Autodesk Inventor part; units mm, degrees
(part 5 of 11)
  arc A1597 (6.6453, 29.3854) -> (6.7017, 29.3342) centre (6.6735, 29.3598) ccw
  line L798 (7.1127, 29.843) -> (7.6112, 30.2647)
  arc A1598 (7.6358, 30.2356) -> (7.5866, 30.2938) centre (7.6112, 30.2647) ccw
  arc A1599 (7.0881, 29.8721) -> (7.1373, 29.8139) centre (7.1127, 29.843) ccw
  line L799 (7.6112, 30.2647) -> (8.1605, 30.6178)
  arc A1600 (8.1811, 30.5857) -> (8.1399, 30.6498) centre (8.1605, 30.6178) ccw
  arc A1601 (7.5906, 30.2968) -> (7.6318, 30.2327) centre (7.6112, 30.2647) ccw
  line L800 (8.1605, 30.6178) -> (8.7512, 30.8961)
  arc A1602 (8.7674, 30.8616) -> (8.7349, 30.9305) centre (8.7511, 30.8961) ccw
  arc A1603 (8.1443, 30.6522) -> (8.1768, 30.5833) centre (8.1605, 30.6178) ccw
  line L801 (8.7512, 30.8961) -> (9.3731, 31.0949)
  arc A1604 (9.3847, 31.0586) -> (9.3615, 31.1312) centre (9.3731, 31.0949) ccw
  arc A1605 (8.7395, 30.9324) -> (8.7627, 30.8598) centre (8.7511, 30.8961) ccw
  line L802 (9.3731, 31.0949) -> (10.0157, 31.2112)
  arc A1606 (10.0224, 31.1737) -> (10.0089, 31.2487) centre (10.0157, 31.2112) ccw
  arc A1607 (9.3663, 31.1324) -> (9.3798, 31.0574) centre (9.3731, 31.0949) ccw
  line L803 (10.0157, 31.2112) -> (10.6676, 31.2441)
  arc A1608 (10.6694, 31.206) -> (10.6658, 31.2821) centre (10.6676, 31.2441) ccw
  arc A1609 (10.0138, 31.2493) -> (10.0175, 31.1731) centre (10.0157, 31.2112) ccw
  line L804 (10.6676, 31.2441) -> (11.2768, 31.2186)
  arc A1610 (11.2731, 31.1809) -> (11.2777, 31.257) centre (11.2754, 31.2189) ccw
  arc A1611 (10.6699, 31.2821) -> (10.6653, 31.2061) centre (10.6676, 31.2441) ccw
  line L805 (11.2768, 31.2186) -> (11.8753, 31.0912)
  arc A1612 (11.8769, 31.0569) -> (11.8906, 31.1319) centre (11.8837, 31.0944) ccw
  arc A1613 (11.2822, 31.2564) -> (11.2685, 31.1815) centre (11.2754, 31.2189) ccw
  line L806 (11.8753, 31.0912) -> (12.4777, 30.9778)
  arc A1614 (12.4664, 30.9414) -> (12.489, 31.0142) centre (12.4777, 30.9778) ccw
  arc A1615 (11.8867, 31.1275) -> (11.864, 31.0548) centre (11.8753, 31.0912) ccw
  line L807 (12.4777, 30.9778) -> (12.9624, 30.6072)
  arc A1616 (12.9467, 30.5724) -> (12.978, 30.6419) centre (12.9624, 30.6072) ccw
  arc A1617 (12.4933, 31.0126) -> (12.462, 30.9431) centre (12.4777, 30.9778) ccw
  line L808 (12.9624, 30.6072) -> (14.3509, 26.7983)
  arc A1618 (14.3312, 26.7657) -> (14.3707, 26.8309) centre (14.3509, 26.7983) ccw
  arc A1619 (12.9821, 30.6398) -> (12.9427, 30.5746) centre (12.9624, 30.6072) ccw
  line L809 (14.3509, 26.7983) -> (23.3981, 15.1516)
  arc A1620 (23.4282, 15.1749) -> (23.4216, 15.1816) centre (23.3981, 15.1516) ccw
  arc A1621 (14.3744, 26.8283) -> (14.3274, 26.7683) centre (14.3509, 26.7983) ccw
  line L810 (23.3981, 15.1516) -> (19.5097, 19.7125)
  arc A1622 (16.8769, 22.7269) -> (16.8787, 22.7253) centre (16.8517, 22.6983) ccw
  arc A1623 (23.3654, 15.132) -> (23.3711, 15.1246) centre (23.3981, 15.1516) ccw
  line L811 (19.5097, 19.7125) -> (16.4438, 23.1565)
  arc A1624 (16.4139, 23.1331) -> (16.4738, 23.18) centre (16.4438, 23.1565) ccw
  arc A1625 (16.8233, 22.673) -> (16.8217, 22.6748) centre (16.8517, 22.6983) ccw
  line L812 (16.4438, 23.1565) -> (16.0942, 23.6606)
  arc A1626 (16.0616, 23.6409) -> (16.1268, 23.6803) centre (16.0942, 23.6606) ccw
  arc A1627 (16.4765, 23.1763) -> (16.4112, 23.1368) centre (16.4438, 23.1565) ccw
  line L813 (16.0942, 23.6606) -> (15.8078, 24.2031)
  arc A1628 (15.7731, 24.1874) -> (15.8426, 24.2187) centre (15.8078, 24.2031) ccw
  arc A1629 (16.1289, 23.6762) -> (16.0594, 23.6449) centre (16.0942, 23.6606) ccw
  line L814 (15.8078, 24.2031) -> (15.5889, 24.7761)
  arc A1630 (15.5525, 24.7648) -> (15.6253, 24.7875) centre (15.5889, 24.7761) ccw
  arc A1631 (15.8442, 24.2144) -> (15.7714, 24.1917) centre (15.8078, 24.2031) ccw
  line L815 (15.5889, 24.7761) -> (15.4407, 25.3714)
  arc A1632 (15.4032, 25.3645) -> (15.4781, 25.3783) centre (15.4407, 25.3714) ccw
  arc A1633 (15.6379, 27.3846) -> (15.5629, 27.3709) centre (15.6004, 27.3777) ccw
  line L816 (15.4407, 25.3714) -> (14.9039, 25.4351)
  arc A1634 (14.8659, 25.4328) -> (14.942, 25.4374) centre (14.9039, 25.4351) ccw
  arc A1635 (15.4787, 25.3737) -> (15.4026, 25.3691) centre (15.4407, 25.3714) ccw
  line L817 (14.9039, 25.4351) -> (18.8583, 22.6449)
  arc A1636 (18.8203, 22.6472) -> (18.8963, 22.6426) centre (18.8583, 22.6449) ccw
  arc A1637 (14.942, 25.4328) -> (14.8659, 25.4374) centre (14.9039, 25.4351) ccw
  line L818 (18.8583, 22.6449) -> (13.5985, 27.0666)
  arc A1638 (15.5629, 24.9531) -> (15.6379, 24.9394) centre (15.6004, 24.9463) ccw
  arc A1639 (18.8958, 22.638) -> (18.8208, 22.6517) centre (18.8583, 22.6449) ccw
  line L819 (13.5985, 27.0666) -> (5.328, 28.9324)
  arc A1640 (5.2916, 28.9437) -> (5.3643, 28.9211) centre (5.328, 28.9324) ccw
  arc A1641 (13.6349, 27.0553) -> (13.5621, 27.0779) centre (13.5985, 27.0666) ccw
  line L820 (5.328, 28.9324) -> (19.749, 27.0115)
  arc A1642 (5.9013, 28.867) -> (5.9708, 28.8358) centre (5.936, 28.8514) ccw
  arc A1643 (5.3627, 28.9167) -> (5.2932, 28.948) centre (5.328, 28.9324) ccw
  line L821 (19.749, 27.0115) -> (10.434, 29.4468)
  arc A1644 (10.4014, 29.4665) -> (10.4666, 29.4271) centre (10.434, 29.4468) ccw
  arc A1645 (19.7816, 26.9918) -> (19.7164, 27.0312) centre (19.749, 27.0115) ccw
  line L822 (10.434, 29.4468) -> (20.7175, 25.3208)
  arc A1646 (10.9892, 29.183) -> (11.0176, 29.2538) centre (11.0034, 29.2184) ccw
  arc A1647 (10.464, 29.4233) -> (10.404, 29.4703) centre (10.434, 29.4468) ccw
  line L823 (20.7175, 25.3208) -> (12.0354, 22.6782)
  arc A1648 (12.0377, 22.6402) -> (12.0332, 22.7163) centre (12.0354, 22.6782) ccw
  arc A1649 (11.0303, 29.1914) -> (10.9764, 29.2453) centre (11.0034, 29.2184) ccw
  line L824 (12.0354, 22.6782) -> (14.4431, 22.5281)
  arc A1650 (14.4196, 22.5581) -> (14.4666, 22.4982) centre (14.4431, 22.5281) ccw
  arc A1651 (12.0589, 22.6482) -> (12.0119, 22.7082) centre (12.0354, 22.6782) ccw
  line L825 (14.4431, 22.5281) -> (13.0207, 21.6798)
  arc A1652 (13.001, 21.7124) -> (13.0404, 21.6472) centre (13.0207, 21.6798) ccw
  arc A1653 (14.4628, 22.4955) -> (14.4234, 22.5608) centre (14.4431, 22.5281) ccw
  line L826 (13.0207, 21.6798) -> (12.4691, 21.4111)
  arc A1654 (12.4535, 21.4459) -> (12.4848, 21.3764) centre (12.4691, 21.4111) ccw
  arc A1655 (13.0363, 21.645) -> (13.005, 21.7145) centre (13.0207, 21.6798) ccw
  line L827 (12.4691, 21.4111) -> (11.8832, 21.2297)
  arc A1656 (11.8719, 21.2661) -> (11.8946, 21.1933) centre (11.8832, 21.2297) ccw
  arc A1657 (12.4805, 21.3748) -> (12.4578, 21.4475) centre (12.4691, 21.4111) ccw
  line L828 (11.8832, 21.2297) -> (11.28, 21.1185)
  arc A1658 (11.2731, 21.156) -> (11.2868, 21.081) centre (11.28, 21.1185) ccw
  arc A1659 (11.8906, 21.1921) -> (11.8769, 21.2671) centre (11.8837, 21.2296) ccw
  line L829 (11.28, 21.1185) -> (10.668, 21.0819)
  arc A1660 (10.6657, 21.1199) -> (10.6703, 21.0439) centre (10.668, 21.0819) ccw
  arc A1661 (11.2823, 21.0805) -> (11.2777, 21.1565) centre (11.28, 21.1185) ccw
  line L830 (10.668, 21.0819) -> (10.0106, 21.1406)
  arc A1662 (10.014, 21.1786) -> (10.0072, 21.1027) centre (10.0106, 21.1406) ccw
  arc A1663 (10.6646, 21.044) -> (10.6714, 21.1199) centre (10.668, 21.0819) ccw
  line L831 (10.0106, 21.1406) -> (9.3659, 21.2818)
  arc A1664 (9.3741, 21.319) -> (9.3578, 21.2446) centre (9.3659, 21.2818) ccw
  arc A1665 (10.0025, 21.1034) -> (10.0188, 21.1778) centre (10.0106, 21.1406) ccw
  line L832 (9.3659, 21.2818) -> (8.7436, 21.502)
  arc A1666 (8.7565, 21.5379) -> (8.7308, 21.4661) centre (8.7436, 21.502) ccw
  arc A1667 (9.3532, 21.2459) -> (9.3787, 21.3177) centre (9.3659, 21.2818) ccw
  line L833 (8.7436, 21.502) -> (8.1556, 21.8016)
  arc A1668 (8.1727, 21.8355) -> (8.1383, 21.7675) centre (8.1555, 21.8015) ccw
  arc A1669 (8.7264, 21.468) -> (8.7608, 21.536) centre (8.7436, 21.502) ccw
  line L834 (8.1556, 21.8016) -> (7.6091, 22.1716)
  arc A1670 (7.6305, 22.2032) -> (7.5877, 22.1401) centre (7.6091, 22.1716) ccw
  arc A1671 (8.1341, 21.7699) -> (8.1768, 21.833) centre (8.1555, 21.8015) ccw
  line L835 (7.6091, 22.1716) -> (7.1138, 22.6078)
  arc A1672 (7.139, 22.6364) -> (7.0887, 22.5793) centre (7.1138, 22.6078) ccw
  arc A1673 (7.5839, 22.143) -> (7.6343, 22.2002) centre (7.6091, 22.1716) ccw
  line L836 (7.1138, 22.6078) -> (6.6776, 23.1031)
  arc A1674 (6.7062, 23.1283) -> (6.649, 23.0779) centre (6.6776, 23.1031) ccw
  arc A1675 (7.0853, 22.5827) -> (7.1424, 22.633) centre (7.1138, 22.6078) ccw
  line L837 (6.6776, 23.1031) -> (6.3075, 23.6495)
  arc A1676 (6.339, 23.6708) -> (6.2759, 23.6281) centre (6.3075, 23.6495) ccw
  arc A1677 (6.6461, 23.0817) -> (6.7092, 23.1245) centre (6.6776, 23.1031) ccw
  line L838 (6.3075, 23.6495) -> (6.0093, 24.2382)
  arc A1678 (6.0432, 24.2554) -> (5.9753, 24.221) centre (6.0093, 24.2382) ccw
  arc A1679 (6.2735, 23.6323) -> (6.3415, 23.6667) centre (6.3075, 23.6495) ccw
  line L839 (6.0093, 24.2382) -> (5.7878, 24.8599)
  arc A1680 (5.8237, 24.8727) -> (5.7519, 24.8472) centre (5.7878, 24.8599) ccw
  arc A1681 (5.9734, 24.2254) -> (6.0451, 24.251) centre (6.0093, 24.2382) ccw
  line L840 (5.7878, 24.8599) -> (5.6466, 25.5046)
  arc A1682 (5.6838, 25.5128) -> (5.6094, 25.4965) centre (5.6466, 25.5046) ccw
  arc A1683 (5.7506, 24.8518) -> (5.825, 24.8681) centre (5.7878, 24.8599) ccw
  line L841 (5.6466, 25.5046) -> (5.588, 26.162)
  arc A1684 (5.6259, 26.1654) -> (5.5501, 26.1586) centre (5.588, 26.162) ccw
  arc A1685 (5.6087, 25.5012) -> (5.6846, 25.508) centre (5.6466, 25.5046) ccw
  line L842 (5.588, 26.162) -> (6.858, 26.162)
  arc A1686 (6.858, 26.1239) -> (6.858, 26.2001) centre (6.858, 26.162) ccw
  arc A1687 (5.588, 26.2001) -> (5.588, 26.1239) centre (5.588, 26.162) ccw
  line L843 (6.858, 26.162) -> (6.8774, 25.6365)
  arc A1688 (6.8393, 25.6351) -> (6.9155, 25.638) centre (6.8774, 25.6366) ccw
  arc A1689 (6.8961, 26.1634) -> (6.8199, 26.1606) centre (6.858, 26.162) ccw
  line L844 (6.8774, 25.6365) -> (6.9714, 25.1192)
  arc A1690 (6.9339, 25.1124) -> (7.0089, 25.126) centre (6.9714, 25.1192) ccw
  arc A1691 (6.9149, 25.6434) -> (6.8399, 25.6297) centre (6.8774, 25.6366) ccw
  line L845 (6.9714, 25.1192) -> (7.1381, 24.6205)
  arc A1692 (7.1019, 24.6085) -> (7.1742, 24.6326) centre (7.1381, 24.6206) ccw
  arc A1693 (7.0075, 25.1313) -> (6.9353, 25.1072) centre (6.9714, 25.1192) ccw
  line L846 (7.1381, 24.6205) -> (7.374, 24.1506)
  arc A1694 (7.34, 24.1335) -> (7.4081, 24.1677) centre (7.374, 24.1506) ccw
  arc A1695 (7.1721, 24.6376) -> (7.104, 24.6035) centre (7.1381, 24.6206) ccw
  line L847 (7.374, 24.1506) -> (7.6744, 23.7191)
  arc A1696 (7.6431, 23.6973) -> (7.7057, 23.7409) centre (7.6744, 23.7191) ccw
  arc A1697 (7.4053, 24.1724) -> (7.3427, 24.1289) centre (7.374, 24.1506) ccw
  line L848 (7.6744, 23.7191) -> (8.0332, 23.3347)
  arc A1698 (8.0053, 23.3087) -> (8.061, 23.3607) centre (8.0332, 23.3347) ccw
  arc A1699 (7.7023, 23.7451) -> (7.6465, 23.6931) centre (7.6744, 23.7191) ccw
  line L849 (8.0332, 23.3347) -> (8.443, 23.0053)
  arc A1700 (8.4191, 22.9756) -> (8.4669, 23.035) centre (8.443, 23.0053) ccw
  arc A1701 (8.057, 23.3644) -> (8.0093, 23.305) centre (8.0332, 23.3347) ccw
  line L850 (8.443, 23.0053) -> (8.8955, 22.7376)
  arc A1702 (8.8761, 22.7048) -> (8.9149, 22.7704) centre (8.8955, 22.7376) ccw
  arc A1703 (8.4624, 23.0381) -> (8.4236, 22.9725) centre (8.443, 23.0053) ccw
  line L851 (8.8955, 22.7376) -> (9.3815, 22.537)
  arc A1704 (9.367, 22.5018) -> (9.3961, 22.5722) centre (9.3815, 22.537) ccw
  arc A1705 (8.91, 22.7728) -> (8.881, 22.7024) centre (8.8955, 22.7376) ccw
  line L852 (9.3815, 22.537) -> (9.8911, 22.4076)
  arc A1706 (9.8818, 22.3706) -> (9.9005, 22.4445) centre (9.8911, 22.4076) ccw
  arc A1707 (9.3909, 22.5739) -> (9.3721, 22.5) centre (9.3815, 22.537) ccw
  line L853 (9.8911, 22.4076) -> (10.414, 22.352)
  arc A1708 (10.41, 22.3141) -> (10.418, 22.3899) centre (10.414, 22.352) ccw
  arc A1709 (9.8952, 22.4455) -> (9.8871, 22.3697) centre (9.8911, 22.4076) ccw
  line L854 (10.414, 22.352) -> (10.6681, 22.3519)
  arc A1710 (10.6681, 22.3138) -> (10.6681, 22.39) centre (10.6681, 22.3519) ccw
  arc A1711 (10.414, 22.3901) -> (10.414, 22.3139) centre (10.414, 22.352) ccw
  line L855 (10.6681, 22.3519) -> (11.2103, 22.3905)
  arc A1712 (11.213, 22.3525) -> (11.2076, 22.4285) centre (11.2103, 22.3905) ccw
  arc A1713 (10.6653, 22.3899) -> (10.6708, 22.3139) centre (10.6681, 22.3519) ccw
  line L856 (11.2103, 22.3905) -> (11.7415, 22.5058)
  arc A1714 (11.7496, 22.4686) -> (11.7334, 22.543) centre (11.7415, 22.5058) ccw
  arc A1715 (11.2022, 22.4277) -> (11.2184, 22.3532) centre (11.2103, 22.3905) ccw
  line L857 (11.7415, 22.5058) -> (12.2509, 22.6955)
  arc A1716 (12.264, 22.6606) -> (12.2374, 22.732) centre (12.2507, 22.6963) ccw
  arc A1717 (11.7282, 22.5415) -> (11.7548, 22.4701) centre (11.7415, 22.5058) ccw
  line L858 (12.2509, 22.6955) -> (12.7282, 22.9558)
  arc A1718 (12.7464, 22.9224) -> (12.7099, 22.9893) centre (12.7282, 22.9558) ccw
  arc A1719 (12.2325, 22.7297) -> (12.269, 22.6629) centre (12.2507, 22.6963) ccw
  line L859 (12.7282, 22.9558) -> (12.9175, 23.4562)
  arc A1720 (13.1859, 23.2521) -> (13.1402, 23.3131) centre (13.163, 23.2826) ccw
  arc A1721 (12.7053, 22.9863) -> (12.751, 22.9253) centre (12.7282, 22.9558) ccw
  line L860 (12.9175, 23.4562) -> (13.0355, 23.9868)
  arc A1722 (13.5743, 23.64) -> (13.5205, 23.6939) centre (13.5474, 23.667) ccw
  arc A1723 (13.1361, 23.3095) -> (13.19, 23.2557) centre (13.163, 23.2826) ccw
  line L861 (13.0355, 23.9868) -> (13.0769, 24.5288)
  arc A1724 (13.1074, 24.506) -> (13.0464, 24.5517) centre (13.0769, 24.5288) ccw
  arc A1725 (13.5169, 23.6898) -> (13.5779, 23.6441) centre (13.5474, 23.667) ccw
  line L862 (13.0769, 24.5288) -> (13.0407, 25.0712)
  arc A1726 (14.1671, 24.561) -> (14.1003, 24.5975) centre (14.1337, 24.5793) ccw
  arc A1727 (13.0435, 24.5471) -> (13.1103, 24.5106) centre (13.0769, 24.5288) ccw
  line L863 (13.0407, 25.0712) -> (12.9277, 25.6029)
  arc A1728 (12.9633, 25.5896) -> (12.892, 25.6162) centre (12.9277, 25.6029) ccw
  arc A1729 (14.098, 24.5926) -> (14.1694, 24.566) centre (14.1337, 24.5793) ccw
  line L864 (12.9277, 25.6029) -> (22.6056, 27.554)
  arc A1730 (22.6429, 27.5459) -> (22.5684, 27.5621) centre (22.6056, 27.554) ccw
  arc A1731 (12.8904, 25.611) -> (12.9649, 25.5948) centre (12.9277, 25.6029) ccw
  line L865 (22.6056, 27.554) -> (9.5434, 30.1539)
  arc A1732 (9.5814, 30.1512) -> (9.5054, 30.1566) centre (9.5434, 30.1539) ccw
  arc A1733 (22.5676, 27.5568) -> (22.6436, 27.5513) centre (22.6056, 27.554) ccw
  line L866 (9.5434, 30.1539) -> (9.9852, 30.1292)
  arc A1734 (10.0232, 30.1319) -> (9.9472, 30.1265) centre (9.9852, 30.1292) ccw
  arc A1735 (9.5054, 30.1512) -> (9.5814, 30.1566) centre (9.5434, 30.1539) ccw
  line L867 (9.9852, 30.1292) -> (10.4403, 29.8319)
  arc A1736 (10.4775, 29.84) -> (10.403, 29.8238) centre (10.4403, 29.8319) ccw
  arc A1737 (9.9479, 30.1211) -> (10.0224, 30.1373) centre (9.9852, 30.1292) ccw
  line L868 (10.4403, 29.8319) -> (10.9331, 29.6024)
  arc A1738 (14.1694, 27.758) -> (14.098, 27.7314) centre (14.1337, 27.7447) ccw
  arc A1739 (10.4046, 29.8186) -> (10.476, 29.8452) centre (10.4403, 29.8319) ccw
  line L869 (10.9331, 29.6024) -> (11.4535, 29.4454)
  arc A1740 (11.4869, 29.4637) -> (11.42, 29.4271) centre (11.4535, 29.4454) ccw
  arc A1741 (14.1003, 27.7265) -> (14.1671, 27.763) centre (14.1337, 27.7447) ccw
  line L870 (11.4535, 29.4454) -> (11.991, 29.364)
  arc A1742 (13.5779, 28.6799) -> (13.5169, 28.6342) centre (13.5474, 28.657) ccw
  arc A1743 (11.423, 29.4226) -> (11.484, 29.4682) centre (11.4535, 29.4454) ccw
  line L871 (11.991, 29.364) -> (12.5346, 29.36)
  arc A1744 (13.19, 29.0683) -> (13.1361, 29.0145) centre (13.163, 29.0414) ccw
  arc A1745 (13.5205, 28.6301) -> (13.5743, 28.684) centre (13.5474, 28.657) ccw
  line L872 (12.5346, 29.36) -> (12.7342, 29.3872)
  arc A1746 (12.7571, 29.4177) -> (12.7114, 29.3567) centre (12.7342, 29.3872) ccw
  arc A1747 (13.1402, 29.0109) -> (13.1859, 29.0719) centre (13.163, 29.0414) ccw
  line L873 (12.7342, 29.3872) -> (12.2551, 29.6441)
  arc A1748 (12.269, 29.6611) -> (12.2325, 29.5943) centre (12.2507, 29.6277) ccw
  arc A1749 (12.716, 29.3537) -> (12.7525, 29.4206) centre (12.7342, 29.3872) ccw
  line L874 (12.2551, 29.6441) -> (11.7444, 29.8301)
  arc A1750 (11.7577, 29.8658) -> (11.7311, 29.7945) centre (11.7444, 29.8301) ccw
  arc A1751 (12.2374, 29.592) -> (12.264, 29.6634) centre (12.2507, 29.6277) ccw
  line L875 (11.7444, 29.8301) -> (11.2123, 29.9416)
  arc A1752 (11.2204, 29.9789) -> (11.2042, 29.9044) centre (11.2123, 29.9416) ccw
  arc A1753 (11.7363, 29.7929) -> (11.7525, 29.8674) centre (11.7444, 29.8301) ccw
  line L876 (11.2123, 29.9416) -> (10.6698, 29.9763)
  arc A1754 (10.6726, 30.0143) -> (10.6671, 29.9383) centre (10.6698, 29.9763) ccw
  arc A1755 (11.2096, 29.9036) -> (11.2151, 29.9796) centre (11.2123, 29.9416) ccw
  line L877 (10.6698, 29.9763) -> (10.1821, 29.9523)
  arc A1756 (10.18, 29.9898) -> (10.1831, 29.9137) centre (10.1815, 29.9518) ccw
  arc A1757 (10.6714, 29.9382) -> (10.6683, 30.0144) centre (10.6698, 29.9763) ccw
  line L878 (10.1821, 29.9523) -> (9.7019, 29.8682)
  arc A1758 (9.6953, 29.9058) -> (9.7084, 29.8307) centre (9.7019, 29.8682) ccw
  arc A1759 (10.1881, 29.9142) -> (10.175, 29.9893) centre (10.1815, 29.9518) ccw
  line L879 (9.7019, 29.8682) -> (9.2372, 29.7228)
  arc A1760 (9.2258, 29.7591) -> (9.2486, 29.6864) centre (9.2372, 29.7228) ccw
  arc A1761 (9.7133, 29.8318) -> (9.6905, 29.9046) centre (9.7019, 29.8682) ccw
  line L880 (9.2372, 29.7228) -> (8.7955, 29.518)
  arc A1762 (8.7795, 29.5525) -> (8.8116, 29.4834) centre (8.7955, 29.5179) ccw
  arc A1763 (9.2533, 29.6882) -> (9.2212, 29.7573) centre (9.2372, 29.7228) ccw
  line L881 (8.7955, 29.518) -> (8.3843, 29.2572)
  arc A1764 (8.3639, 29.2894) -> (8.4047, 29.225) centre (8.3843, 29.2572) ccw
  arc A1765 (8.8159, 29.4857) -> (8.7751, 29.5501) centre (8.7955, 29.5179) ccw
  line L882 (8.3843, 29.2572) -> (8.0107, 28.945)
  arc A1766 (7.9863, 28.9742) -> (8.0352, 28.9157) centre (8.0107, 28.945) ccw
  arc A1767 (8.4088, 29.228) -> (8.3599, 29.2864) centre (8.3843, 29.2572) ccw
  line L883 (8.0107, 28.945) -> (7.6811, 28.5867)
  arc A1768 (7.653, 28.6125) -> (7.7091, 28.5609) centre (7.6811, 28.5867) ccw
  arc A1769 (8.0388, 28.9192) -> (7.9827, 28.9708) centre (8.0107, 28.945) ccw
  line L884 (7.6811, 28.5867) -> (7.401, 28.1884)
  arc A1770 (7.3698, 28.2104) -> (7.4321, 28.1665) centre (7.401, 28.1884) ccw
  arc A1771 (7.7122, 28.5648) -> (7.6499, 28.6086) centre (7.6811, 28.5867) ccw
  line L885 (7.401, 28.1884) -> (7.1753, 27.757)
  arc A1772 (7.1415, 27.7747) -> (7.209, 27.7394) centre (7.1753, 27.757) ccw
  arc A1773 (7.4347, 28.1708) -> (7.3672, 28.2061) centre (7.401, 28.1884) ccw
  line L886 (7.1753, 27.757) -> (7.6204, 27.5599)
  arc A1774 (6.972, 27.313) -> (7.0436, 27.2868) centre (7.0078, 27.2999) ccw
  arc A1775 (7.211, 27.7439) -> (7.1395, 27.7702) centre (7.1753, 27.757) ccw
  line L887 (7.6204, 27.5599) -> (6.9014, 26.8247)
  arc A1776 (6.8642, 26.8331) -> (6.9386, 26.8164) centre (6.9014, 26.8247) ccw
  arc A1777 (12.9568, 32.9698) -> (12.8825, 32.9865) centre (12.9197, 32.9781) ccw
  line L888 (6.9014, 26.8247) -> (6.858, 26.3398)
  arc A1778 (6.8201, 26.3432) -> (6.8959, 26.3364) centre (6.858, 26.3398) ccw
  arc A1779 (6.9394, 26.8213) -> (6.8635, 26.8281) centre (6.9014, 26.8247) ccw
  line L889 (6.858, 26.3398) -> (5.588, 26.3398)
  arc A1780 (5.588, 26.3779) -> (5.588, 26.3017) centre (5.588, 26.3398) ccw
  arc A1781 (6.858, 26.3017) -> (6.858, 26.3779) centre (6.858, 26.3398) ccw
  line L890 (15.4591, 25.2973) -> (14.7422, 26.1051)
  arc A1782 (14.7041, 26.1051) -> (14.7803, 26.1051) centre (14.7422, 26.1051) ccw
  arc A1783 (15.4972, 25.2973) -> (15.421, 25.2973) centre (15.4591, 25.2973) ccw
  line L891 (15.6556, 24.6016) -> (14.6713, 26.8246)
  arc A1784 (14.6332, 26.8246) -> (14.7094, 26.8246) centre (14.6713, 26.8246) ccw
  arc A1785 (15.6937, 24.6016) -> (15.6175, 24.6016) centre (15.6556, 24.6016) ccw
  line L892 (15.8368, 24.1482) -> (5.3895, 28.9242)
  arc A1786 (5.3514, 28.9242) -> (5.4276, 28.9242) centre (5.3895, 28.9242) ccw
  arc A1787 (15.8749, 24.1482) -> (15.7987, 24.1482) centre (15.8368, 24.1482) ccw
  line L893 (16.0101, 23.8198) -> (14.7162, 27.6819)
  arc A1788 (14.6781, 27.6819) -> (14.7543, 27.6819) centre (14.7162, 27.6819) ccw
  arc A1789 (16.0482, 23.8198) -> (15.972, 23.8198) centre (16.0101, 23.8198) ccw
  line L894 (16.1807, 23.5359) -> (19.6022, 27.0499)
  arc A1790 (19.5641, 27.0499) -> (19.6403, 27.0499) centre (19.6022, 27.0499) ccw
  arc A1791 (16.2188, 23.5359) -> (16.1426, 23.5359) centre (16.1807, 23.5359) ccw
  line L895 (16.3486, 23.2938) -> (14.8395, 28.295)
  arc A1792 (14.8014, 28.295) -> (14.8776, 28.295) centre (14.8395, 28.295) ccw
  arc A1793 (16.3867, 23.2938) -> (16.3105, 23.2938) centre (16.3486, 23.2938) ccw
  line L896 (16.515, 23.0767) -> (16.1422, 29.0049)
  arc A1794 (16.1041, 29.0049) -> (16.1803, 29.0049) centre (16.1422, 29.0049) ccw
  arc A1795 (16.5531, 23.0767) -> (16.4769, 23.0767) centre (16.515, 23.0767) ccw
  line L897 (16.6793, 22.8921) -> (10.7626, 29.315)
  arc A1796 (10.7245, 29.315) -> (10.8007, 29.315) centre (10.7626, 29.315) ccw
  arc A1797 (16.7174, 22.8921) -> (16.6412, 22.8921) centre (16.6793, 22.8921) ccw
  line L898 (12.0171, 28.1294) -> (9.5434, 30.1539)
  arc A1798 (9.5053, 30.1539) -> (9.5815, 30.1539) centre (9.5434, 30.1539) ccw
  arc A1799 (12.0552, 28.1294) -> (11.979, 28.1294) centre (12.0171, 28.1294) ccw
  line L899 (9.5434, 30.1539) -> (9.9028, 29.66)
  arc A1800 (9.8647, 29.66) -> (9.9409, 29.66) centre (9.9028, 29.66) ccw
  arc A1801 (9.5815, 30.1539) -> (9.5053, 30.1539) centre (9.5434, 30.1539) ccw
  line L900 (19.6426, 19.5567) -> (10.4327, 29.8369)
  arc A1802 (10.3946, 29.8369) -> (10.4708, 29.8369) centre (10.4327, 29.8369) ccw
  arc A1803 (19.6807, 19.5567) -> (19.6045, 19.5567) centre (19.6426, 19.5567) ccw
  line L901 (21.7522, 27.382) -> (20.5215, 25.2612)
  arc A1804 (20.4834, 25.2612) -> (20.5596, 25.2612) centre (20.5215, 25.2612) ccw
  arc A1805 (21.7903, 27.382) -> (21.7141, 27.382) centre (21.7522, 27.382) ccw
  line L902 (12.3669, 28.0907) -> (10.8306, 29.6501)
  arc A1806 (10.7925, 29.6501) -> (10.8687, 29.6501) centre (10.8306, 29.6501) ccw
  arc A1807 (12.405, 28.0907) -> (12.3288, 28.0907) centre (12.3669, 28.0907) ccw
  line L903 (13.0172, 25.1818) -> (14.192, 23.3346)
  arc A1808 (14.1539, 23.3346) -> (14.2301, 23.3346) centre (14.192, 23.3346) ccw
  arc A1809 (13.0553, 25.1818) -> (12.9791, 25.1818) centre (13.0172, 25.1818) ccw
  line L904 (12.58, 28.0916) -> (11.1586, 29.5344)
  arc A1810 (11.1205, 29.5344) -> (11.1967, 29.5344) centre (11.1586, 29.5344) ccw
  arc A1811 (12.6181, 28.0916) -> (12.5419, 28.0916) centre (12.58, 28.0916) ccw
  line L905 (13.0564, 24.8362) -> (14.1433, 23.1272)
  arc A1812 (14.1052, 23.1272) -> (14.1814, 23.1272) centre (14.1433, 23.1272) ccw
  arc A1813 (13.0945, 24.8362) -> (13.0183, 24.8362) centre (13.0564, 24.8362) ccw
  line L906 (23.5292, 14.9828) -> (11.4614, 29.4442)
  arc A1814 (11.4233, 29.4442) -> (11.4995, 29.4442) centre (11.4614, 29.4442) ccw
  arc A1815 (23.5673, 14.9828) -> (23.4911, 14.9828) centre (23.5292, 14.9828) ccw
  line L907 (13.0763, 24.5209) -> (12.2488, 22.6649)
  arc A1816 (12.2107, 22.6649) -> (12.2869, 22.6649) centre (12.2488, 22.6649) ccw
  arc A1817 (13.1144, 24.5209) -> (13.0382, 24.5209) centre (13.0763, 24.5209) ccw
  line L908 (23.648, 14.8299) -> (11.7128, 29.4061)
  arc A1818 (11.6747, 29.4061) -> (11.7509, 29.4061) centre (11.7128, 29.4061) ccw
  arc A1819 (23.6861, 14.8299) -> (23.6099, 14.8299) centre (23.648, 14.8299) ccw
  line L909 (13.0569, 24.2673) -> (12.442, 22.6529)
  arc A1820 (12.4039, 22.6529) -> (12.4801, 22.6529) centre (12.442, 22.6529) ccw
  arc A1821 (13.095, 24.2673) -> (13.0188, 24.2673) centre (13.0569, 24.2673) ccw
  line L910 (13.278, 28.1796) -> (11.9643, 29.3681)
  arc A1822 (11.9262, 29.3681) -> (12.0024, 29.3681) centre (11.9643, 29.3681) ccw
  arc A1823 (13.3161, 28.1796) -> (13.2399, 28.1796) centre (13.278, 28.1796) ccw
  line L911 (13.0376, 24.0137) -> (13.9419, 22.5594)
  arc A1824 (13.9038, 22.5594) -> (13.98, 22.5594) centre (13.9419, 22.5594) ccw
  arc A1825 (13.0757, 24.0137) -> (12.9995, 24.0137) centre (13.0376, 24.0137) ccw
  line L912 (14.2939, 26.9548) -> (13.2686, 25.6803)
  arc A1826 (13.2305, 25.6803) -> (13.3067, 25.6803) centre (13.2686, 25.6803) ccw
  arc A1827 (14.332, 26.9548) -> (14.2558, 26.9548) centre (14.2939, 26.9548) ccw
  line L913 (14.3098, 24.0785) -> (14.3, 22.4428)
  arc A1828 (14.2619, 22.4428) -> (14.3381, 22.4428) centre (14.3, 22.4428) ccw
  arc A1829 (14.3479, 24.0785) -> (14.2717, 24.0785) centre (14.3098, 24.0785) ccw
  line L914 (14.2329, 27.1221) -> (13.2454, 25.8946)
  arc A1830 (13.2073, 25.8946) -> (13.2835, 25.8946) centre (13.2454, 25.8946) ccw
  arc A1831 (14.271, 27.1221) -> (14.1948, 27.1221) centre (14.2329, 27.1221) ccw
  line L915 (14.1565, 23.927) -> (14.1471, 22.3516)
  arc A1832 (14.109, 22.3516) -> (14.1852, 22.3516) centre (14.1471, 22.3516) ccw
  arc A1833 (14.1946, 23.927) -> (14.1184, 23.927) centre (14.1565, 23.927) ccw
  line L916 (13.7852, 28.3501) -> (12.6046, 29.3695)
  arc A1834 (12.5665, 29.3695) -> (12.6427, 29.3695) centre (12.6046, 29.3695) ccw
  arc A1835 (13.8233, 28.3501) -> (13.7471, 28.3501) centre (13.7852, 28.3501) ccw
  line L917 (12.8925, 23.39) -> (13.6973, 22.0834)
  arc A1836 (13.6592, 22.0834) -> (13.7354, 22.0834) centre (13.6973, 22.0834) ccw
  arc A1837 (12.9306, 23.39) -> (12.8544, 23.39) centre (12.8925, 23.39) ccw
  line L918 (12.8972, 30.657) -> (12.5563, 29.2005)
  arc A1838 (12.5182, 29.2005) -> (12.5944, 29.2005) centre (12.5563, 29.2005) ccw
  arc A1839 (12.9353, 30.657) -> (12.8591, 30.657) centre (12.8972, 30.657) ccw
  line L919 (12.9015, 23.1391) -> (12.9469, 21.6439)
  arc A1840 (12.9088, 21.6439) -> (12.985, 21.6439) centre (12.9469, 21.6439) ccw
  arc A1841 (12.9396, 23.1391) -> (12.8634, 23.1391) centre (12.9015, 23.1391) ccw
  line L920 (12.7645, 30.7585) -> (12.4339, 29.3463)
  arc A1842 (12.3958, 29.3463) -> (12.472, 29.3463) centre (12.4339, 29.3463) ccw
  arc A1843 (12.8026, 30.7585) -> (12.7264, 30.7585) centre (12.7645, 30.7585) ccw
  line L921 (12.7526, 23.0204) -> (12.7967, 21.5707)
  arc A1844 (12.7586, 21.5707) -> (12.8348, 21.5707) centre (12.7967, 21.5707) ccw
  arc A1845 (12.7907, 23.0204) -> (12.7145, 23.0204) centre (12.7526, 23.0204) ccw
  line L922 (12.6444, 30.8503) -> (12.6553, 29.4295)
  arc A1846 (12.6172, 29.4295) -> (12.6934, 29.4295) centre (12.6553, 29.4295) ccw
  arc A1847 (12.6825, 30.8503) -> (12.6063, 30.8503) centre (12.6444, 30.8503) ccw
  line L923 (12.6495, 22.9129) -> (12.6464, 21.4975)
  arc A1848 (12.6083, 21.4975) -> (12.6845, 21.4975) centre (12.6464, 21.4975) ccw
  arc A1849 (12.6876, 22.9129) -> (12.6114, 22.9129) centre (12.6495, 22.9129) ccw
  line L924 (12.4915, 30.9178) -> (12.5022, 29.5116)
  arc A1850 (12.4641, 29.5116) -> (12.5403, 29.5116) centre (12.5022, 29.5116) ccw
  arc A1851 (12.5296, 30.9178) -> (12.4534, 30.9178) centre (12.4915, 30.9178) ccw
  line L925 (12.4971, 22.8298) -> (12.4962, 21.4243)
  arc A1852 (12.4581, 21.4243) -> (12.5343, 21.4243) centre (12.4962, 21.4243) ccw
  arc A1853 (12.5352, 22.8298) -> (12.459, 22.8298) centre (12.4971, 22.8298) ccw
  line L926 (12.3387, 30.9679) -> (12.3492, 29.5936)
  arc A1854 (12.3111, 29.5936) -> (12.3873, 29.5936) centre (12.3492, 29.5936) ccw
  arc A1855 (12.3768, 30.9679) -> (12.3006, 30.9679) centre (12.3387, 30.9679) ccw
  line L927 (12.3446, 22.7466) -> (12.344, 21.3723)
  arc A1856 (12.3059, 21.3723) -> (12.3821, 21.3723) centre (12.344, 21.3723) ccw
  arc A1857 (12.3827, 22.7466) -> (12.3065, 22.7466) centre (12.3446, 22.7466) ccw
  line L928 (12.1921, 31.0316) -> (12.1963, 29.6655)
  arc A1858 (12.1582, 29.6655) -> (12.2344, 29.6655) centre (12.1963, 29.6655) ccw
  arc A1859 (12.2302, 31.0316) -> (12.154, 31.0316) centre (12.1921, 31.0316) ccw
  line L929 (12.1922, 22.6736) -> (12.1916, 21.3252)
  arc A1860 (12.1535, 21.3252) -> (12.2297, 21.3252) centre (12.1916, 21.3252) ccw
  arc A1861 (12.2303, 22.6736) -> (12.1541, 22.6736) centre (12.1922, 22.6736) ccw
  line L930 (12.0334, 31.0614) -> (12.0434, 29.7212)
  arc A1862 (12.0053, 29.7212) -> (12.0815, 29.7212) centre (12.0434, 29.7212) ccw
  arc A1863 (12.0715, 31.0614) -> (11.9953, 31.0614) centre (12.0334, 31.0614) ccw
  line L931 (12.0398, 22.6169) -> (12.039, 21.2779)
  arc A1864 (12.0009, 21.2779) -> (12.0771, 21.2779) centre (12.039, 21.2779) ccw
  arc A1865 (12.0779, 22.6169) -> (12.0017, 22.6169) centre (12.0398, 22.6169) ccw
  line L932 (11.8805, 31.1069) -> (11.8906, 29.7769)
  arc A1866 (11.8525, 29.7769) -> (11.9287, 29.7769) centre (11.8906, 29.7769) ccw
  arc A1867 (11.9186, 31.1069) -> (11.8424, 31.1069) centre (11.8805, 31.1069) ccw
  line L933 (11.8874, 22.5601) -> (11.8867, 21.2301)
  arc A1868 (11.8486, 21.2301) -> (11.9248, 21.2301) centre (11.8867, 21.2301) ccw
  arc A1869 (11.9255, 22.5601) -> (11.8493, 22.5601) centre (11.8874, 22.5601) ccw
  line L934 (11.7348, 31.1217) -> (11.7348, 29.8191)
  arc A1870 (11.6967, 29.8191) -> (11.7729, 29.8191) centre (11.7348, 29.8191) ccw
  arc A1871 (11.7729, 31.1217) -> (11.6967, 31.1217) centre (11.7348, 31.1217) ccw
  line L935 (11.7348, 22.5049) -> (11.7348, 21.2023)
  arc A1872 (11.6967, 21.2023) -> (11.7729, 21.2023) centre (11.7348, 21.2023) ccw
  arc A1873 (11.7729, 22.5049) -> (11.6967, 22.5049) centre (11.7348, 22.5049) ccw
  line L936 (11.5757, 31.155) -> (11.5851, 29.8635)
  arc A1874 (11.547, 29.8635) -> (11.6232, 29.8635) centre (11.5851, 29.8635) ccw
  arc A1875 (11.6138, 31.155) -> (11.5376, 31.155) centre (11.5757, 31.155) ccw
  line L937 (11.5825, 22.4713) -> (11.582, 21.1742)
  arc A1876 (11.5439, 21.1742) -> (11.6201, 21.1742) centre (11.582, 21.1742) ccw
  arc A1877 (11.6206, 22.4713) -> (11.5444, 22.4713) centre (11.5825, 22.4713) ccw
  line L938 (11.4226, 31.1876) -> (11.4325, 29.8955)
  arc A1878 (11.3944, 29.8955) -> (11.4706, 29.8955) centre (11.4325, 29.8955) ccw
  arc A1879 (11.4607, 31.1876) -> (11.3845, 31.1876) centre (11.4226, 31.1876) ccw
  line L939 (11.4301, 22.4382) -> (11.4295, 21.1461)
  arc A1880 (11.3914, 21.1461) -> (11.4676, 21.1461) centre (11.4295, 21.1461) ccw
  arc A1881 (11.4682, 22.4382) -> (11.392, 22.4382) centre (11.4301, 22.4382) ccw
  line L940 (11.27, 31.214) -> (11.2798, 29.9275)
  arc A1882 (11.2417, 29.9275) -> (11.3179, 29.9275) centre (11.2798, 29.9275) ccw
  arc A1883 (11.3081, 31.214) -> (11.2319, 31.214) centre (11.27, 31.214) ccw
  line L941 (11.2777, 22.4051) -> (11.2771, 21.1186)
  arc A1884 (11.239, 21.1186) -> (11.3152, 21.1186) centre (11.2771, 21.1186) ccw
  arc A1885 (11.3158, 22.4051) -> (11.2396, 22.4051) centre (11.2777, 22.4051) ccw
  line L942 (11.1215, 31.2251) -> (11.1453, 29.9503)
  arc A1886 (11.1072, 29.9503) -> (11.1834, 29.9503) centre (11.1453, 29.9503) ccw
  arc A1887 (11.1596, 31.2251) -> (11.0834, 31.2251) centre (11.1215, 31.2251) ccw
  line L943 (11.1258, 22.3843) -> (11.1249, 21.1092)
  arc A1888 (11.0868, 21.1092) -> (11.163, 21.1092) centre (11.1249, 21.1092) ccw
  arc A1889 (11.1639, 22.3843) -> (11.0877, 22.3843) centre (11.1258, 22.3843) ccw
  line L944 (10.969, 31.2315) -> (10.9748, 29.9568)
  arc A1890 (10.9367, 29.9568) -> (11.0129, 29.9568) centre (10.9748, 29.9568) ccw
  arc A1891 (11.0071, 31.2315) -> (10.9309, 31.2315) centre (10.969, 31.2315) ccw
  line L945 (10.9729, 22.3736) -> (10.9725, 21.1001)
  arc A1892 (10.9344, 21.1001) -> (11.0106, 21.1001) centre (10.9725, 21.1001) ccw
  arc A1893 (11.011, 22.3736) -> (10.9348, 22.3736) centre (10.9729, 22.3736) ccw
  line L946 (10.8126, 31.238) -> (10.8223, 29.9665)
  arc A1894 (10.7842, 29.9665) -> (10.8604, 29.9665) centre (10.8223, 29.9665) ccw
  arc A1895 (10.8507, 31.238) -> (10.7745, 31.238) centre (10.8126, 31.238) ccw
  line L947 (10.8205, 22.3628) -> (10.8198, 21.091)
  arc A1896 (10.7817, 21.091) -> (10.8579, 21.091) centre (10.8198, 21.091) ccw
  arc A1897 (10.8586, 22.3628) -> (10.7824, 22.3628) centre (10.8205, 22.3628) ccw
  line L948 (10.6676, 31.2441) -> (10.6698, 29.9763)
  arc A1898 (10.6317, 29.9763) -> (10.7079, 29.9763) centre (10.6698, 29.9763) ccw
  arc A1899 (10.7057, 31.2441) -> (10.6295, 31.2441) centre (10.6676, 31.2441) ccw
  line L949 (10.6681, 22.3519) -> (10.668, 21.0819)
  arc A1900 (10.6299, 21.0819) -> (10.7061, 21.0819) centre (10.668, 21.0819) ccw
  arc A1901 (10.7062, 22.3519) -> (10.63, 22.352) centre (10.6681, 22.3519) ccw
  line L950 (10.5152, 31.2364) -> (10.5175, 29.9688)
  arc A1902 (10.4794, 29.9688) -> (10.5556, 29.9688) centre (10.5175, 29.9688) ccw
  arc A1903 (10.5533, 31.2364) -> (10.4771, 31.2364) centre (10.5152, 31.2364) ccw
  line L951 (10.5157, 22.352) -> (10.5156, 21.0955)
  arc A1904 (10.4775, 21.0955) -> (10.5537, 21.0955) centre (10.5156, 21.0955) ccw
  arc A1905 (10.5538, 22.352) -> (10.4776, 22.352) centre (10.5157, 22.352) ccw
  line L952 (10.3629, 31.2287) -> (10.3651, 29.9613)
  arc A1906 (10.327, 29.9613) -> (10.4032, 29.9613) centre (10.3651, 29.9613) ccw
  arc A1907 (10.401, 31.2287) -> (10.3248, 31.2287) centre (10.3629, 31.2287) ccw
  line L953 (10.3633, 22.3574) -> (10.3632, 21.1091)
  arc A1908 (10.3251, 21.1091) -> (10.4013, 21.1091) centre (10.3632, 21.1091) ccw
  arc A1909 (10.4014, 22.3574) -> (10.3252, 22.3574) centre (10.3633, 22.3574) ccw
  line L954 (10.2105, 31.221) -> (10.2142, 29.9538)
  arc A1910 (10.1761, 29.9538) -> (10.2523, 29.9538) centre (10.2142, 29.9538) ccw
  arc A1911 (10.2486, 31.221) -> (10.1724, 31.221) centre (10.2105, 31.221) ccw
  line L955 (10.2108, 22.3736) -> (10.2108, 21.1228)
  arc A1912 (10.1727, 21.1228) -> (10.2489, 21.1228) centre (10.2108, 21.1228) ccw
  arc A1913 (10.2489, 22.3736) -> (10.1727, 22.3736) centre (10.2108, 22.3736) ccw
  line L956 (10.0579, 31.2133) -> (10.059, 29.9307)
  arc A1914 (10.0209, 29.9307) -> (10.0971, 29.9307) centre (10.059, 29.9307) ccw
  arc A1915 (10.096, 31.2133) -> (10.0198, 31.2133) centre (10.0579, 31.2133) ccw
  line L957 (10.0584, 22.3898) -> (10.0584, 21.1364)
  arc A1916 (10.0203, 21.1364) -> (10.0965, 21.1364) centre (10.0584, 21.1364) ccw
  arc A1917 (10.0965, 22.3898) -> (10.0203, 22.3898) centre (10.0584, 22.3898) ccw
  line L958 (9.9059, 31.1913) -> (9.9066, 29.904)
  arc A1918 (9.8685, 29.904) -> (9.9447, 29.904) centre (9.9066, 29.904) ccw
  arc A1919 (9.944, 31.1913) -> (9.8678, 31.1913) centre (9.9059, 31.1913) ccw
  line L959 (9.906, 22.406) -> (9.906, 21.1635)
  arc A1920 (9.8679, 21.1635) -> (9.9441, 21.1635) centre (9.906, 21.1635) ccw
  arc A1921 (9.9441, 22.406) -> (9.8679, 22.406) centre (9.906, 22.406) ccw
  line L960 (9.7535, 31.1637) -> (9.7542, 29.8774)
  arc A1922 (9.7161, 29.8774) -> (9.7923, 29.8774) centre (9.7542, 29.8774) ccw
  arc A1923 (9.7916, 31.1637) -> (9.7154, 31.1637) centre (9.7535, 31.1637) ccw
  line L961 (9.7536, 22.4425) -> (9.7536, 21.1969)
  arc A1924 (9.7155, 21.1969) -> (9.7917, 21.1969) centre (9.7536, 21.1969) ccw
  arc A1925 (9.7917, 22.4425) -> (9.7155, 22.4425) centre (9.7536, 22.4425) ccw
  line L962 (9.6011, 31.1362) -> (9.6012, 29.8367)
  arc A1926 (9.5631, 29.8367) -> (9.6393, 29.8367) centre (9.6012, 29.8367) ccw
  arc A1927 (9.6392, 31.1362) -> (9.563, 31.1362) centre (9.6011, 31.1362) ccw
  line L963 (9.6012, 22.4812) -> (9.6012, 21.2303)
  arc A1928 (9.5631, 21.2303) -> (9.6393, 21.2303) centre (9.6012, 21.2303) ccw
  arc A1929 (9.6393, 22.4812) -> (9.5631, 22.4812) centre (9.6012, 22.4812) ccw
  line L964 (9.4488, 31.1086) -> (9.4488, 29.789)
  arc A1930 (9.4107, 29.789) -> (9.4869, 29.789) centre (9.4488, 29.789) ccw
  arc A1931 (9.4869, 31.1086) -> (9.4107, 31.1086) centre (9.4488, 31.1086) ccw
  line L965 (9.4488, 22.5199) -> (9.4488, 21.2637)
  arc A1932 (9.4107, 21.2637) -> (9.4869, 21.2637) centre (9.4488, 21.2637) ccw
  arc A1933 (9.4869, 22.5199) -> (9.4107, 22.5199) centre (9.4488, 22.5199) ccw
  line L966 (9.2963, 31.0703) -> (9.2964, 29.7413)
  arc A1934 (9.2583, 29.7413) -> (9.3345, 29.7413) centre (9.2964, 29.7413) ccw
  arc A1935 (9.3344, 31.0703) -> (9.2582, 31.0703) centre (9.2963, 31.0703) ccw
  line L967 (9.2935, 22.572) -> (9.2962, 21.3065)
  arc A1936 (9.2581, 21.3065) -> (9.3343, 21.3065) centre (9.2962, 21.3065) ccw
  arc A1937 (9.3316, 22.572) -> (9.2554, 22.572) centre (9.2935, 22.572) ccw
  line L968 (9.144, 31.0217) -> (9.144, 29.6795)
  arc A1938 (9.1059, 29.6795) -> (9.1821, 29.6795) centre (9.144, 29.6795) ccw
  arc A1939 (9.1821, 31.0217) -> (9.1059, 31.0217) centre (9.144, 31.0217) ccw
  line L969 (9.144, 22.635) -> (9.1437, 21.3604)
  arc A1940 (9.1056, 21.3604) -> (9.1818, 21.3604) centre (9.1437, 21.3604) ccw
  arc A1941 (9.1821, 22.635) -> (9.1059, 22.635) centre (9.144, 22.635) ccw
  line L970 (8.9917, 30.973) -> (8.9916, 29.6089)
  arc A1942 (8.9535, 29.6089) -> (9.0297, 29.6089) centre (8.9916, 29.6089) ccw
  arc A1943 (9.0298, 30.973) -> (8.9536, 30.973) centre (8.9917, 30.973) ccw
  line L971 (8.9885, 22.6972) -> (8.9912, 21.4144)
  arc A1944 (8.9531, 21.4144) -> (9.0293, 21.4144) centre (8.9912, 21.4144) ccw
  arc A1945 (9.0266, 22.6972) -> (8.9504, 22.6972) centre (8.9885, 22.6972) ccw
  line L972 (8.8391, 30.9242) -> (8.8392, 29.5382)
  arc A1946 (8.8011, 29.5382) -> (8.8773, 29.5382) centre (8.8392, 29.5382) ccw
  arc A1947 (8.8772, 30.9242) -> (8.801, 30.9242) centre (8.8391, 30.9242) ccw
  line L973 (8.8392, 22.7709) -> (8.8392, 21.4694)
  arc A1948 (8.8011, 21.4694) -> (8.8773, 21.4694) centre (8.8392, 21.4694) ccw
  arc A1949 (8.8773, 22.7709) -> (8.8011, 22.7709) centre (8.8392, 22.7709) ccw
  line L974 (8.6868, 30.8657) -> (8.6868, 29.449)
  arc A1950 (8.6487, 29.449) -> (8.7249, 29.449) centre (8.6868, 29.449) ccw
  arc A1951 (8.7249, 30.8657) -> (8.6487, 30.8657) centre (8.6868, 30.8657) ccw
  line L975 (8.6868, 22.8611) -> (8.6863, 21.5312)
  arc A1952 (8.6482, 21.5312) -> (8.7244, 21.5312) centre (8.6863, 21.5312) ccw
  arc A1953 (8.7249, 22.8611) -> (8.6487, 22.8611) centre (8.6868, 22.8611) ccw
  line L976 (8.5343, 30.7939) -> (8.5344, 29.3523)
  arc A1954 (8.4963, 29.3523) -> (8.5725, 29.3523) centre (8.5344, 29.3523) ccw
  arc A1955 (8.5724, 30.7939) -> (8.4962, 30.7939) centre (8.5343, 30.7939) ccw
  line L977 (8.5344, 22.9512) -> (8.5344, 21.6096)
  arc A1956 (8.4963, 21.6096) -> (8.5725, 21.6096) centre (8.5344, 21.6096) ccw
  arc A1957 (8.5725, 22.9512) -> (8.4963, 22.9512) centre (8.5344, 22.9512) ccw
  line L978 (8.3819, 30.7221) -> (8.382, 29.2552)
  arc A1958 (8.3439, 29.2552) -> (8.4201, 29.2552) centre (8.382, 29.2552) ccw
  arc A1959 (8.42, 30.7221) -> (8.3438, 30.7221) centre (8.3819, 30.7221) ccw
  line L979 (8.382, 23.0543) -> (8.3818, 21.6863)
  arc A1960 (8.3437, 21.6863) -> (8.4199, 21.6863) centre (8.3818, 21.6863) ccw
  arc A1961 (8.4201, 23.0543) -> (8.3439, 23.0543) centre (8.382, 23.0543) ccw
  line L980 (8.2296, 30.6503) -> (8.2296, 29.1279)
  arc A1962 (8.1915, 29.1279) -> (8.2677, 29.1279) centre (8.2296, 29.1279) ccw
  arc A1963 (8.2677, 30.6503) -> (8.1915, 30.6503) centre (8.2296, 30.6503) ccw
  line L981 (8.2296, 23.1768) -> (8.2296, 21.7639)
  arc A1964 (8.1915, 21.7639) -> (8.2677, 21.7639) centre (8.2296, 21.7639) ccw
  arc A1965 (8.2677, 23.1768) -> (8.1915, 23.1768) centre (8.2296, 23.1768) ccw
  line L982 (8.0772, 30.5642) -> (8.0772, 29.0005)
  arc A1966 (8.0391, 29.0005) -> (8.1153, 29.0005) centre (8.0772, 29.0005) ccw
  arc A1967 (8.1153, 30.5642) -> (8.0391, 30.5642) centre (8.0772, 30.5642) ccw
  line L983 (8.0772, 23.2993) -> (8.0773, 21.8546)
  arc A1968 (8.0392, 21.8546) -> (8.1154, 21.8546) centre (8.0773, 21.8546) ccw
  arc A1969 (8.1153, 23.2993) -> (8.0391, 23.2993) centre (8.0772, 23.2993) ccw
  line L984 (7.9248, 30.4662) -> (7.9248, 28.8516)
  arc A1970 (7.8867, 28.8516) -> (7.9629, 28.8516) centre (7.9248, 28.8516) ccw
  arc A1971 (7.9629, 30.4662) -> (7.8867, 30.4662) centre (7.9248, 30.4662) ccw
  line L985 (7.9248, 23.4508) -> (7.9249, 21.9578)
  arc A1972 (7.8868, 21.9578) -> (7.963, 21.9578) centre (7.9249, 21.9578) ccw
  arc A1973 (7.9629, 23.4508) -> (7.8867, 23.4508) centre (7.9248, 23.4508) ccw
  line L986 (7.7724, 30.3683) -> (7.7724, 28.6859)
  arc A1974 (7.7343, 28.6859) -> (7.8105, 28.6859) centre (7.7724, 28.6859) ccw
  arc A1975 (7.8105, 30.3683) -> (7.7343, 30.3683) centre (7.7724, 30.3683) ccw
  line L987 (7.7724, 23.6141) -> (7.7724, 22.061)
  arc A1976 (7.7343, 22.061) -> (7.8105, 22.061) centre (7.7724, 22.061) ccw
  arc A1977 (7.8105, 23.6141) -> (7.7343, 23.6141) centre (7.7724, 23.6141) ccw
  line L988 (7.62, 30.2703) -> (7.62, 28.4999)
  arc A1978 (7.5819, 28.4999) -> (7.6581, 28.4999) centre (7.62, 28.4999) ccw
  arc A1979 (7.6581, 30.2703) -> (7.5819, 30.2703) centre (7.62, 30.2703) ccw
  line L989 (7.62, 23.7973) -> (7.62, 22.1642)
  arc A1980 (7.5819, 22.1642) -> (7.6581, 22.1642) centre (7.62, 22.1642) ccw
  arc A1981 (7.6581, 23.7973) -> (7.5819, 23.7973) centre (7.62, 23.7973) ccw
  line L990 (7.4676, 30.1432) -> (7.4676, 28.2832)
  arc A1982 (7.4295, 28.2832) -> (7.5057, 28.2832) centre (7.4676, 28.2832) ccw
  arc A1983 (7.5057, 30.1432) -> (7.4295, 30.1432) centre (7.4676, 30.1432) ccw
  line L991 (7.4676, 24.0162) -> (7.4676, 22.2963)
  arc A1984 (7.4295, 22.2963) -> (7.5057, 22.2963) centre (7.4676, 22.2963) ccw
  arc A1985 (7.5057, 24.0162) -> (7.4295, 24.0162) centre (7.4676, 24.0162) ccw
  line L992 (7.3152, 30.0143) -> (7.3152, 28.0245)
  arc A1986 (7.2771, 28.0245) -> (7.3533, 28.0245) centre (7.3152, 28.0245) ccw
  arc A1987 (7.3533, 30.0143) -> (7.2771, 30.0143) centre (7.3152, 30.0143) ccw
  line L993 (7.3152, 24.2678) -> (7.3152, 22.4305)
  arc A1988 (7.2771, 22.4305) -> (7.3533, 22.4305) centre (7.3152, 22.4305) ccw
  arc A1989 (7.3533, 24.2678) -> (7.2771, 24.2678) centre (7.3152, 24.2678) ccw
  line L994 (7.1628, 29.8854) -> (7.2084, 27.7423)
  arc A1990 (7.1703, 27.7423) -> (7.2465, 27.7423) centre (7.2084, 27.7423) ccw
  arc A1991 (7.2009, 29.8854) -> (7.1247, 29.8854) centre (7.1628, 29.8854) ccw
  line L995 (7.1628, 24.5713) -> (7.1628, 22.5647)
  arc A1992 (7.1247, 22.5647) -> (7.2009, 22.5647) centre (7.1628, 22.5647) ccw
  arc A1993 (7.2009, 24.5713) -> (7.1247, 24.5713) centre (7.1628, 24.5713) ccw
  line L996 (7.0104, 29.7304) -> (7.6135, 27.563)
  arc A1994 (7.5754, 27.563) -> (7.6516, 27.563) centre (7.6135, 27.563) ccw
  arc A1995 (7.0485, 29.7304) -> (6.9723, 29.7304) centre (7.0104, 29.7304) ccw
  line L997 (7.0104, 25.0026) -> (7.0104, 22.7253)
  arc A1996 (6.9723, 22.7253) -> (7.0485, 22.7253) centre (7.0104, 22.7253) ccw
  arc A1997 (7.0485, 25.0026) -> (6.9723, 25.0026) centre (7.0104, 25.0026) ccw
  line L998 (6.858, 29.5628) -> (6.858, 26.3398)
  arc A1998 (6.8199, 26.3398) -> (6.8961, 26.3398) centre (6.858, 26.3398) ccw
  arc A1999 (6.8961, 29.5628) -> (6.8199, 29.5628) centre (6.858, 29.5628) ccw
  line L999 (6.858, 26.162) -> (6.858, 22.8983)
  arc A2000 (6.8199, 22.8983) -> (6.8961, 22.8983) centre (6.858, 22.8983) ccw
  arc A2001 (6.8961, 26.162) -> (6.8199, 26.162) centre (6.858, 26.162) ccw
  line L1000 (6.7056, 29.3951) -> (6.7056, 26.3398)
  arc A2002 (6.6675, 26.3398) -> (6.7437, 26.3398) centre (6.7056, 26.3398) ccw
  arc A2003 (6.7437, 29.3951) -> (6.6675, 29.3951) centre (6.7056, 29.3951) ccw
  line L1001 (6.7056, 26.162) -> (6.7056, 23.0713)
  arc A2004 (6.6675, 23.0713) -> (6.7437, 23.0713) centre (6.7056, 23.0713) ccw
  arc A2005 (6.7437, 26.162) -> (6.6675, 26.162) centre (6.7056, 26.162) ccw
  line L1002 (6.5532, 29.1865) -> (6.5532, 26.3398)
  arc A2006 (6.5151, 26.3398) -> (6.5913, 26.3398) centre (6.5532, 26.3398) ccw
  arc A2007 (6.5913, 29.1865) -> (6.5151, 29.1865) centre (6.5532, 29.1865) ccw
  line L1003 (6.5532, 26.162) -> (6.5532, 23.2868)
  arc A2008 (6.5151, 23.2868) -> (6.5913, 23.2868) centre (6.5532, 23.2868) ccw
  arc A2009 (6.5913, 26.162) -> (6.5151, 26.162) centre (6.5532, 26.162) ccw
  line L1004 (6.4008, 28.967) -> (6.4008, 26.3398)
  arc A2010 (6.3627, 26.3398) -> (6.4389, 26.3398) centre (6.4008, 26.3398) ccw
  arc A2011 (6.4389, 28.967) -> (6.3627, 28.967) centre (6.4008, 28.967) ccw
  line L1005 (6.4008, 26.162) -> (6.4008, 23.5117)
  arc A2012 (6.3627, 23.5117) -> (6.4389, 23.5117) centre (6.4008, 23.5117) ccw
  arc A2013 (6.4389, 26.162) -> (6.3627, 26.162) centre (6.4008, 26.162) ccw
  line L1006 (6.2484, 28.7212) -> (6.2484, 26.3398)
  arc A2014 (6.2103, 26.3398) -> (6.2865, 26.3398) centre (6.2484, 26.3398) ccw
  arc A2015 (6.2865, 28.7212) -> (6.2103, 28.7212) centre (6.2484, 28.7212) ccw
  line L1007 (6.2484, 26.162) -> (6.2484, 23.7661)
  arc A2016 (6.2103, 23.7661) -> (6.2865, 23.7661) centre (6.2484, 23.7661) ccw
  arc A2017 (6.2865, 26.162) -> (6.2103, 26.162) centre (6.2484, 26.162) ccw
  line L1008 (6.096, 28.4255) -> (6.096, 26.3398)
  arc A2018 (6.0579, 26.3398) -> (6.1341, 26.3398) centre (6.096, 26.3398) ccw
  arc A2019 (6.1341, 28.4255) -> (6.0579, 28.4255) centre (6.096, 28.4255) ccw
  line L1009 (6.096, 26.162) -> (6.096, 24.067)
  arc A2020 (6.0579, 24.067) -> (6.1341, 24.067) centre (6.096, 24.067) ccw
  arc A2021 (6.1341, 26.162) -> (6.0579, 26.162) centre (6.096, 26.162) ccw
  line L1010 (5.9436, 28.0807) -> (5.9436, 26.3398)
  arc A2022 (5.9055, 26.3398) -> (5.9817, 26.3398) centre (5.9436, 26.3398) ccw
  arc A2023 (5.9817, 28.0807) -> (5.9055, 28.0807) centre (5.9436, 28.0807) ccw
  line L1011 (5.9436, 26.162) -> (5.9436, 24.4226)
  arc A2024 (5.9055, 24.4226) -> (5.9817, 24.4226) centre (5.9436, 24.4226) ccw
  arc A2025 (5.9817, 26.162) -> (5.9055, 26.162) centre (5.9436, 26.162) ccw
  line L1012 (5.7912, 27.6567) -> (5.7912, 26.3398)
  arc A2026 (5.7531, 26.3398) -> (5.8293, 26.3398) centre (5.7912, 26.3398) ccw
  arc A2027 (5.8293, 27.6567) -> (5.7531, 27.6567) centre (5.7912, 27.6567) ccw
  line L1013 (5.7912, 26.162) -> (5.7912, 24.8504)
  arc A2028 (5.7531, 24.8504) -> (5.8293, 24.8504) centre (5.7912, 24.8504) ccw
  arc A2029 (5.8293, 26.162) -> (5.7531, 26.162) centre (5.7912, 26.162) ccw
  line L1014 (5.6388, 26.9485) -> (5.6388, 26.3398)
  arc A2030 (5.6007, 26.3398) -> (5.6769, 26.3398) centre (5.6388, 26.3398) ccw
  arc A2031 (5.6769, 26.9485) -> (5.6007, 26.9485) centre (5.6388, 26.9485) ccw
  line L1015 (5.6388, 26.162) -> (5.6388, 25.5924)
  arc A2032 (5.6007, 25.5924) -> (5.6769, 25.5924) centre (5.6388, 25.5924) ccw
  arc A2033 (5.6769, 26.162) -> (5.6007, 26.162) centre (5.6388, 26.162) ccw
  line L1016 (28.3443, 10.7495) -> (31.1877, 9.8395)
  arc A2034 (31.1497, 9.8426) -> (31.2257, 9.8363) centre (31.1877, 9.8395) ccw
  arc A2035 (28.3823, 10.7463) -> (28.3063, 10.7527) centre (28.3443, 10.7495) ccw
  line L1017 (31.1877, 9.8395) -> (31.0489, 9.2014)
  arc A2036 (31.0117, 9.2095) -> (31.0861, 9.1933) centre (31.0489, 9.2014) ccw
  arc A2037 (31.2249, 9.8314) -> (31.1505, 9.8476) centre (31.1877, 9.8395) ccw
  line L1018 (31.0489, 9.2014) -> (30.8281, 8.5869)
  arc A2038 (30.7922, 8.5998) -> (30.8639, 8.5741) centre (30.828, 8.5869) ccw
  arc A2039 (31.0848, 9.1885) -> (31.0131, 9.2143) centre (31.0489, 9.2014) ccw
  line L1019 (30.8281, 8.5869) -> (30.5289, 8.0066)
  arc A2040 (30.495, 8.024) -> (30.5627, 7.9891) centre (30.5289, 8.0066) ccw
  arc A2041 (30.8619, 8.5695) -> (30.7942, 8.6044) centre (30.8281, 8.5869) ccw
  line L1020 (30.5289, 8.0066) -> (30.1565, 7.4702)
  arc A2042 (30.1252, 7.4919) -> (30.1878, 7.4484) centre (30.1565, 7.4702) ccw
  arc A2043 (30.5602, 7.9848) -> (30.4976, 8.0283) centre (30.5289, 8.0065) ccw
  line L1021 (30.1565, 7.4702) -> (29.7173, 6.987)
  arc A2044 (29.6891, 7.0126) -> (29.7455, 6.9614) centre (29.7173, 6.987) ccw
  arc A2045 (30.1847, 7.4446) -> (30.1283, 7.4958) centre (30.1565, 7.4702) ccw
  line L1022 (29.7173, 6.987) -> (29.2188, 6.5653)
  arc A2046 (29.1942, 6.5944) -> (29.2434, 6.5362) centre (29.2188, 6.5653) ccw
  arc A2047 (29.7419, 6.9579) -> (29.6927, 7.0161) centre (29.7173, 6.987) ccw
  line L1023 (29.2188, 6.5653) -> (28.6694, 6.2122)
  arc A2048 (28.6489, 6.2443) -> (28.6901, 6.1802) centre (28.6694, 6.2122) ccw
  arc A2049 (29.2394, 6.5332) -> (29.1982, 6.5973) centre (29.2188, 6.5653) ccw
  line L1024 (28.6694, 6.2122) -> (28.0788, 5.9339)
  arc A2050 (28.0649, 5.9692) -> (28.0963, 5.8997) centre (28.0806, 5.9344) ccw
  arc A2051 (28.6857, 6.1778) -> (28.6532, 6.2467) centre (28.6694, 6.2122) ccw
  line L1025 (28.0788, 5.9339) -> (27.4548, 5.7455)
  arc A2052 (27.4439, 5.782) -> (27.4671, 5.7094) centre (27.4555, 5.7457) ccw
  arc A2053 (28.0922, 5.8981) -> (28.069, 5.9707) centre (28.0806, 5.9344) ccw
  line L1026 (27.4548, 5.7455) -> (26.8144, 5.6169)
  arc A2054 (26.8078, 5.6544) -> (26.8213, 5.5794) centre (26.8146, 5.6169) ccw
  arc A2055 (27.4623, 5.7082) -> (27.4487, 5.7832) centre (27.4555, 5.7457) ccw
  line L1027 (26.8144, 5.6169) -> (26.1621, 5.5887)
  arc A2056 (26.1603, 5.6267) -> (26.1639, 5.5506) centre (26.1621, 5.5887) ccw
  arc A2057 (26.8164, 5.5789) -> (26.8128, 5.655) centre (26.8146, 5.6169) ccw
  line L1028 (26.1621, 5.5887) -> (25.5497, 5.6254)
  arc A2058 (25.552, 5.6634) -> (25.5474, 5.5874) centre (25.5497, 5.6254) ccw
  arc A2059 (26.1598, 5.5506) -> (26.1644, 5.6267) centre (26.1621, 5.5887) ccw
  line L1029 (25.5497, 5.6254) -> (24.9463, 5.7358)
  arc A2060 (24.9531, 5.7731) -> (24.9394, 5.6981) centre (24.9463, 5.7356) ccw
  arc A2061 (25.5429, 5.588) -> (25.5566, 5.6629) centre (25.5497, 5.6254) ccw
  line L1030 (24.9463, 5.7358) -> (24.3605, 5.918)
  arc A2062 (24.3718, 5.9544) -> (24.3492, 5.8816) centre (24.3605, 5.918) ccw
  arc A2063 (24.935, 5.6994) -> (24.9576, 5.7721) centre (24.9463, 5.7358) ccw
  line L1031 (24.3605, 5.918) -> (23.8011, 6.1698)
  arc A2064 (23.8168, 6.2045) -> (23.7855, 6.1351) centre (23.8011, 6.1698) ccw